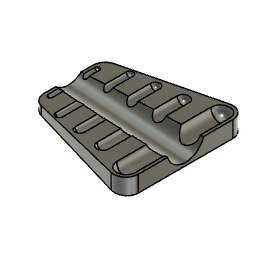
CenterDrillTray (Autodesk Fusion 360 design; units mm, degrees)
Autodesk Fusion 360 part; units mm, degrees
other "Base Mesh Feature1"
sketch "Sketch1" plane through (0, 0, 19) normal (0, 0, 1) x (1, 0, 0)
  line L0 (-33.1125, 0) -> (45.8125, 0) construction
  line L1 (-27.9375, -15.875) -> (-27.9375, 15.875)
  arc A0 (-27.9375, 15.875) -> (-31.1125, 15.875) centre (-29.525, 15.875) ccw
  line L2 (-31.1125, 15.875) -> (-31.1125, -15.875)
  arc A1 (-31.1125, -15.875) -> (-27.9375, -15.875) centre (-29.525, -15.875) ccw
  line L3 (-29.525, -17.4625) -> (-29.525, 17.4625)
  line L4 (-13.175, -23.8125) -> (-13.175, 23.8125)
  arc A2 (-13.175, 23.8125) -> (-17.9375, 23.8125) centre (-15.5562, 23.8125) ccw
  line L5 (-17.9375, 23.8125) -> (-17.9375, -23.8125)
  arc A3 (-17.9375, -23.8125) -> (-13.175, -23.8125) centre (-15.5562, -23.8125) ccw
  line L6 (-15.5562, -26.1937) -> (-15.5562, 26.1937)
  line L7 (3.175, -25.4) -> (3.175, 25.4)
  arc A4 (3.175, 25.4) -> (-3.175, 25.4) centre (0, 25.4) ccw
  line L8 (-3.175, 25.4) -> (-3.175, -25.4)
  arc A5 (-3.175, -25.4) -> (3.175, -25.4) centre (0, -25.4) ccw
  line L9 (0, -28.575) -> (0, 28.575)
  line L10 (21.1125, -26.9875) -> (21.1125, 26.9875)
  arc A6 (21.1125, 26.9875) -> (13.175, 26.9875) centre (17.1438, 26.9875) ccw
  line L11 (13.175, 26.9875) -> (13.175, -26.9875)
  arc A7 (13.175, -26.9875) -> (21.1125, -26.9875) centre (17.1438, -26.9875) ccw
  line L12 (17.1438, -30.9563) -> (17.1438, 30.9563)
  line L13 (43.8125, -31.75) -> (43.8125, 31.75)
  arc A8 (43.8125, 31.75) -> (31.1125, 31.75) centre (37.4625, 31.75) ccw
  line L14 (31.1125, 31.75) -> (31.1125, -31.75)
  arc A9 (31.1125, -31.75) -> (43.8125, -31.75) centre (37.4625, -31.75) ccw
  line L15 (37.4625, -38.1) -> (37.4625, 38.1)
  line L16 (-27.9375, 15.875) -> (-17.9375, 15.875) construction
  line L17 (-13.175, 21.8743) -> (-3.175, 21.8743) construction
  line L18 (13.175, 21.8742) -> (3.175, 21.8742) construction
  line L19 (21.1125, -39.1242) -> (31.1125, -39.1242) construction
  line L20 (-33.1125, 0) -> (-33.1125, 22.9719)
  line L21 (-33.1125, 22.9719) -> (45.8125, 42.4054)
  line L22 (45.8125, 42.4054) -> (45.8125, 0)
  line L23 (43.8125, 31.75) -> (45.8125, 31.75) construction
  line L24 (-31.1125, 15.875) -> (-33.1125, 15.875) construction
  line L25 (-33.1125, -22.9719) -> (45.8125, -42.4054)
  line L26 (-33.1125, 0) -> (-33.1125, -22.9719)
  line L27 (45.8125, -42.4054) -> (45.8125, 0)
  circle A10 centre (37.4625, 31.75) radius 8.35 construction
  line L28 (-16.1256, 26.1247) -> (-16.3647, 27.0957) construction
  point P0 (-29.525, 0)
  point P1 (-15.5562, 0)
  point P2 (17.1438, 0)
  point P3 (37.4625, 0)
  dimension "d1" = 3.175
  dimension "d2" = 4.7625
  dimension "d3" = 6.35
  dimension "d4" = 7.9375
  dimension "d5" = 12.7
  dimension "d6" = 31.75
  dimension "d7" = 47.625
  dimension "d8" = 50.8
  dimension "d9" = 63.5
  dimension "d10" = 2
  dimension "d11" = 10
  dimension "d12" = 1
  dimension "d13" = 53.975
  constraint horizontal L0
  constraint tangent L1 A0
  constraint tangent A0 L2
  constraint parallel L1 L2
  constraint tangent L2 A1
  constraint tangent L1 A1
  constraint perpendicular L0 L3
  constraint coincident L0 P0
  constraint tangent L4 A2
  constraint tangent A2 L5
  constraint parallel L4 L5
  constraint tangent L5 A3
  constraint tangent L4 A3
  constraint perpendicular L0 L6
  constraint coincident L0 P1
  constraint tangent L7 A4
  constraint tangent A4 L8
  constraint parallel L7 L8
  constraint tangent L8 A5
  constraint tangent L7 A5
  constraint perpendicular L0 L9
  constraint coincident L0 origin
  constraint tangent L10 A6
  constraint tangent A6 L11
  constraint parallel L10 L11
  constraint tangent L11 A7
  constraint tangent L10 A7
  constraint perpendicular L0 L12
  constraint coincident L0 P2
  constraint tangent L13 A8
  constraint tangent A8 L14
  constraint parallel L13 L14
  constraint tangent L14 A9
  constraint tangent L13 A9
  constraint perpendicular L0 L15
  constraint coincident L0 P3
  constraint coincident L5 L16.end
  constraint perpendicular L5 L16
  constraint coincident L4 L17.start
  constraint coincident L8 L17.end
  constraint perpendicular L8 L17
  constraint coincident L11 L18.start
  constraint coincident L7 L18.end
  constraint perpendicular L7 L18
  constraint coincident L10 L19.start
  constraint coincident L14 L19.end
  constraint perpendicular L14 L19
  constraint equal L18 L19
  constraint equal L17 L18
  constraint equal L16 L17
  constraint perpendicular L0 L20
  constraint vertical L22
  constraint coincident L22 L23.end
  constraint perpendicular L22 L23
  constraint coincident L20 L24.end
  constraint perpendicular L20 L24
  constraint equal L23 L24
  constraint symmetric L20.start L0 L26.start
  constraint symmetric L22.end L0 L27.end
  constraint symmetric L0 L20.end L25.start
  constraint symmetric L0 L21.end L25.end
  constraint concentric A8 A10
  constraint tangent L21 A10
  constraint tangent L22 A10
  constraint coincident A2 L28.start
  constraint coincident L21 L28.end
  constraint perpendicular L21 L28
  constraint coincident A2.centre L28
  constraint coincident A0 L3.end
  constraint coincident L3 P0
  constraint coincident A0.centre L3
  constraint coincident A1 L3.start
  constraint coincident A1.centre L3
  constraint coincident A3 L6.start
  constraint coincident L6 P1
  constraint coincident A3.centre L6
  constraint coincident A5 L9.start
  constraint coincident L9 origin
  constraint coincident A5.centre L9
  constraint coincident A7 L12.start
  constraint coincident L12 P2
  constraint coincident A7.centre L12
  constraint coincident A9 L15.start
  constraint coincident L15 P3
  constraint coincident A9.centre L15
  constraint coincident A8 L15.end
  constraint coincident A8.centre L15
  constraint coincident A6 L12.end
  constraint coincident A6.centre L12
  constraint coincident A4 L9.end
  constraint coincident A4.centre L9
  constraint coincident A2 L6.end
  constraint coincident A2.centre L6
  measures "d1" diameter of A0
  measures "d2" diameter of A2
  measures "d3" diameter of A4
  measures "d4" diameter of A6
  measures "d5" diameter of A8
  measures "d6" distance of A1.centre A0.centre
  measures "d7" distance of A3.centre A2.centre
  measures "d8" distance of A5.centre A4.centre
  measures "d9" distance of A9.centre A8.centre
  measures "d10" distance of L13.end L23.end
  measures "d11" distance of L1.end L16.end
  measures "d12" distance of L28.start L28.end
  measures "d13" distance of A7.centre A6.centre
other "MeshSection1"
extrude "Extrude1" add sketch "Sketch1" against normal blind 13.7 contours L1 A0 A1 L3 | A0 L2 A1 L3 | L4 A2 A3 L6 | A2 L5 A3 L6 | L7 A4 A5 L9 | A4 L8 A5 L9 | L10 A6 A7 L12 | A6 L11 A7 L12 | L13 A8 A9 L15 | A8 L14 A9 L15 | L20 L21 L22 L25 L26 L27
revolve "Revolve1" cut sketch "Sketch1" angle 360 about axis through (37.4625, -38.1, 19) along (0, 1, 0) contours A8 L14 A9 L15
revolve "Revolve2" cut sketch "Sketch1" angle 360 about axis through (17.1438, -30.9563, 19) along (0, 1, 0) contours L10 A6 A7 L12
revolve "Revolve3" cut sketch "Sketch1" angle 360 about axis through (0, -28.575, 19) along (0, 1, 0) contours L7 A4 A5 L9
revolve "Revolve4" cut sketch "Sketch1" angle 360 about axis through (-29.525, -17.4625, 19) along (0, 1, 0) contours A0 L2 A1 L3
revolve "Revolve5" cut sketch "Sketch1" angle 360 about axis through (-15.5562, -26.1937, 19) along (0, 1, 0) contours L4 A2 A3 L6
fillet "Fillet1" radius 8.255 4 edges at (45.8125, -42.4054, 12.15) (45.8125, 42.4054, 12.15) (-33.1125, 22.9719, 12.15) (-33.1125, -22.9719, 12.15)
sketch "Sketch2" plane through (0, 0, 0) normal (0, 1, 0) x (1, 0, 0)
  arc A0 (21.1125, -19) -> (13.175, -19) centre (17.1438, -19) ccw
  arc A1 (3.175, -19) -> (-3.175, -19) centre (0, -19) ccw
  arc A2 (-13.175, -19) -> (-17.9375, -19) centre (-15.5562, -19) ccw
  arc A3 (-27.9375, -19) -> (-31.1125, -19) centre (-29.525, -19) ccw
  arc A4 (43.8125, -19) -> (31.1125, -19) centre (37.4625, -19) ccw
  line L0 (45.8125, -19) -> (45.8125, -5.3)
  line L1 (-33.1125, -5.3) -> (-33.1125, -19)
  line L2 (-33.1125, -13.654) -> (45.8125, -8.0286)
  line L3 (37.011, -12.6661) -> (36.7267, -8.6762) construction
  line L4 (-29.6379, -17.4165) -> (-29.9222, -13.4266) construction
  line L5 (-33.1125, -5.3) -> (45.8125, -5.3)
  dimension "d24" = 4
  constraint coincident L1 L2.start
  constraint coincident L0 L2.end
  constraint coincident A4 L3.start
  constraint coincident L2 L3.end
  constraint perpendicular L2 L3
  constraint coincident L2 L4.end
  constraint perpendicular L2 L4
  constraint coincident A3 L4.start
  constraint coincident A3.centre L4
  constraint coincident A4.centre L3
  constraint equal L3 L4
  constraint coincident L1.start L5.start
  constraint coincident L0.end L5.end
  measures "d24" distance of L3.start L3.end
extrude "Extrude2" cut sketch "Sketch2" along normal mid plane 132.08
ref_plane "WorkPlane1" through (47.179, 31.8712, 27.201) normal (0.99747, 0, -0.071095) x (0, 1, 0)
sketch "Sketch3" plane through (47.179, 31.8712, 27.201) normal (0.99747, 0, -0.071095) x (0, 1, 0)
  line L0 (-63.7425, -19.2211) -> (0, -19.2211) construction
  line L1 (0, -19.2211) -> (0, -8.2774) construction
  line L2 (0, -8.2774) -> (-63.7425, -8.2774) construction
  line L3 (-63.7425, -8.2774) -> (-63.7425, -19.2211) construction
  line L4 (-31.8712, -8.2774) -> (-31.8712, -19.2211) construction
  line L5 (-19.1712, -4.5211) -> (-19.1712, -8.2774)
  arc A0 (-19.1712, -8.2774) -> (-44.5712, -8.2774) centre (-31.8712, -8.2774) ccw
  line L6 (-44.5712, -8.2774) -> (-44.5712, -4.5211)
  arc A1 (-44.5712, -4.5211) -> (-19.1712, -4.5211) centre (-31.8712, -4.5211) ccw
  line L7 (-31.8712, -17.2211) -> (-31.8712, 4.4226) construction
  dimension "d27" = 12.7
  dimension "d28" = 2
  constraint midpoint L2 L4.start
  constraint midpoint L0 L4.end
  constraint tangent L5 A0
  constraint tangent A0 L6
  constraint parallel L5 L6
  constraint tangent L6 A1
  constraint tangent L5 A1
  constraint midpoint A1 L7.start
  constraint midpoint A0 L7.end
  constraint perpendicular L2 L7
  constraint coincident L4 L7.start
  constraint coincident L4.start A0.centre
  measures "d27" radius of A0
  measures "d28" distance of L4.end L7.start
extrude "Extrude3" cut sketch "Sketch3" against normal blind 88.9 contours A0 A1
equation "d2 = ( 3 / 16 ) * 1 in"
equation "d4 = ( 5 / 16 ) * 1 in"
equation "d10 = 2 * minT"
equation "minT = 1 mm"
equation "d15 = -0.5 in - minT"
equation "d24 = 4 * minT"
equation "d28 = 2 * minT"
